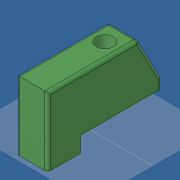
# Autodesk Inventor part: Schalter_Knauf
Saved by Autodesk Inventor 2019 (Build 230136000, 136)
## iProperties
Created: 2020-08-07
Part Number: Schalter_Knauf
Material: Generisch
Document SubType Name: Modeling
Designer: Stefan
Mass: 5.65641 g
Surface Area: 26.5432 cm^2
Volume: 5.65641 cm^3
Density: 1 g/cm^3
Appearance: Glatt - waldgrün
Author: Stefan
Autodesk Inventor part; units mm, degrees
ref_plane "YZ Plane" through (0, 0, 0) normal (1, 0, 0) x (0, 1, 0)
ref_plane "XZ Plane" through (0, 0, 0) normal (0, 1, 0) x (-1, 0, 0)
ref_plane "XY Plane" through (0, 0, 0) normal (0, 0, 1) x (1, 0, 0)
sketch "Skizze1" plane through (0, 0, 0) normal (0, 1, 0) x (-1, 0, 0)
  line L0 (5, 18.5) -> (-5, 18.5)
  line L1 (-5, 18.5) -> (-5, -18.5)
  line L2 (-5, -18.5) -> (5, -18.5)
  line L3 (5, -18.5) -> (5, 18.5)
  line L4 (5, 18.5) -> (-5, -18.5) construction
  line L5 (-5, 18.5) -> (5, -18.5) construction
  circle A0 centre (0, -4.75) radius 13.75 construction
  arc A1 (-5, -17.5587) -> (5, -17.5587) centre (0, -4.75) ccw
  arc A2 (5, 8.0587) -> (-5, 8.0587) centre (0, -4.75) ccw
  line L6 (0, -18.5) -> (0, 9) construction
  circle A3 centre (0, -13.75) radius 1.5
  circle A4 centre (0, 4.25) radius 1.5
  line L7 (-5, -4.75) -> (5, -4.75) construction
  circle A5 centre (0, -13.75) radius 4 construction
  circle A6 centre (0, 4.25) radius 4 construction
  circle A7 centre (0, -4.75) radius 2.75
  point P0 (0, 0)
  point P1 (0, 0)
  dimension "d2" = 37
  dimension "d3" = 10
  dimension "d4" = 27.5
  dimension "d18" = 3
  dimension "d20" = 18
  dimension "d23" = 8
  dimension "d24" = 8
  dimension "d25" = 5.5
  constraints: 16 end point, 10 point on circle, 8 centre point, 8 point on line, 5 midpoint, 3 coincident, 2 equal radius, 2 parallel, 2 perpendicular, 2 tangent, 1 horizontal, 1 symmetric about line, 1 vertical alignment
  measures "d2" distance between parallel lines of L0 L2
  measures "d3" distance between parallel lines of L1 L3
  measures "d4" diameter of A0
  measures "d18" diameter of A3
  measures "d20" distance of A4.centre A3.centre
  measures "d23" diameter of A5
  measures "d24" diameter of A6
  measures "d25" diameter of A7
extrude "Extrusion1" add sketch "Skizze1" along normal blind 22 contours L3 A2 L1 L0 | L3 A1 L1 A2 | A3 | A4
sketch "Skizze2" plane through (0, 0, 0) normal (1, 0, 0) x (0, 1, 0)
  line L0 (0, -18.5) -> (0, -7.5) projected
  line L1 (0, 18.5) -> (22, 18.5) projected
  line L2 (22, -7.5) -> (22, -18.5) projected
  line L3 (7, -18.5) -> (22, -10.5244)
  line L4 (22, -18.5) -> (0, -18.5) projected
  line L5 (22, -10.5244) -> (22, -18.5)
  line L6 (22, -18.5) -> (7, -18.5)
  line L7 (0, -7.5) -> (22, -7.5) projected
  line L8 (22, 18.5) -> (22, -2) projected
  line L9 (22, -2) -> (0, -2) projected
  line L10 (0, -2) -> (0, 18.5) projected
  dimension "d14" = 62
  dimension "d15" = 7
  constraints: 6 end point, 1 perpendicular, 1 point on line, 1 vertical
  measures "d14" angle of L3 L2
  measures "d15" distance of L0.start L3.start
extrude "Extrusion5" cut sketch "Skizze2" along normal through all both and the other way through all contours L3 L2 L4
extrude "Extrusion3" cut sketch "Skizze1" along normal blind 5 contours L3 A1 L1 A2 | L3 L2 A1 | A1 L2 L1 | A3 | A4 | A7
extrude "Extrusion6" cut sketch "Skizze1" along normal blind 11 contours A3 | A4
fillet "Rundung1" radius 1 9 edges at (5, 22, 3.9878) (-5, 22, 3.9878) (0, 22, -10.5244) (5, 15.3852, -14.0415) (5, 6.8852, -17.5587) (-5, 6.8852, -17.5587) (-5, 15.3852, -14.0415) (-5, 11, 18.5) (5, 11, 18.5)
